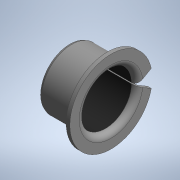
# Autodesk Inventor part: LFF-1410
Saved by Autodesk Inventor 2020.2 (Build 242310000, 310)
## iProperties
Part Number: LFF-1410
Material: 一般
Catalog Web Link: www.cadenas.de
Description: Flange Bushings-LFF
Vendor: OILES
Document SubType Name: Modeling
Designer: partserver
Manufacturer: OILES
Mass: 0.655588 g
Surface Area: 14.435 cm^2
Volume: 0.655588 cm^3
Density: 1 g/cm^3
Appearance: PSOLRGB-175-175-175
Category: PARTsolutions
Company: OILES
PSOL_IDENT_0: {$CADENAS_DATA\23d-libs\oiles\multi_bearings\oiles_drymet_lf\flange_bushings_lff.prj},166 {VTYP=3D},
PSOL_IDENT_1: {NB=LFF-1410},{LINA=LFF-1410},{NN=Flange Bushings},{DATE=15.04.2019 22:54:28},{GEOMDATE=27.10.2016 0
PSOL_IDENT_2: 4:28:40},{VERSION=},{LINEID=630},{WBVAR=},{WBNUMERIC=}  {NB=LFF-1410},{LINA=LFF-1410},{KT=DUMMY},{OR
PSOL_IDENT_3: DERNO=LFF-1410},{S=14},{SRT=-0.025/-0.043},{H=16.0},{HRT=H7(+0.018/0)},{ID=14},{IDR=+0.068/0},{OD=16
PSOL_IDENT_4: .0},{IDT=+0.065/+0.035},{T=1.0},{TT=0/-0.025},{F=22},{R=1.500},{FDT=0/-0.8},{FT=1.0},{FTT=0/-0.15},{
PSOL_IDENT_5: L=10},{LT=0/-0.3},{A=0.5},{AX=0.500},{B=C0.3},{BC=0.300},{TE=-200~+280°C},{P=49.0N/mm2 (500kgf/cm2)}
PSOL_IDENT_6: ,{V=0.65m/s (39m/min)},{PV=3.60N/mm2•m/s (2,200kgf/cm2•m/min)},{AIT=The I.D. tolerance after press f
PSOL_IDENT_7: itting is for reference only.},{AOT=Outer diameter is measrued by exclusive gauge.},{CAU=Please refe
PSOL_IDENT_8: r to catalog about detail.}
NB: LFF-1410
NN: Flange Bushings
NT: LFF
NBSYN: $ORDERNO.
LINA: LFF-1410
CATALOG: OILES CORPORATION
ORDERNO: LFF-1410
S: 14
SRT: -0.025/-0.043
H: 16
HRT: H7(+0.018/0)
ID: 14
IDR: +0.068/0
OD: 16
IDT: +0.065/+0.035
T: 1
TT: 0/-0.025
F: 22
FDT: 0/-0.8
FT: 1
FTT: 0/-0.15
L: 10
LT: 0/-0.3
TE: -200~+280°C
P: 49.0N/mm2 (500kgf/cm2)
V: 0.65m/s (39m/min)
PV: 3.60N/mm2•m/s (2,200kgf/cm2•m/min)
AIT: The I.D. tolerance after press fitting is for reference only.
AOT: Outer diameter is measrued by exclusive gauge.
CAU: Please refer to catalog about detail.
SUPPLIER: OILES
ARTICLENO: LFF-1410
BOMINFO: LFF-1410
CREATOR: CADENAS GmbH
Title: LFF-1410
Author: Cadenas PARTsolutions
Comments: LFF
Autodesk Inventor part; units mm, degrees
ref_plane "YZ Plane" through (0, 0, 0) normal (1, 0, 0) x (0, 1, 0)
ref_plane "XZ Plane" through (0, 0, 0) normal (0, 1, 0) x (-1, 0, 0)
ref_plane "XY Plane" through (0, 0, 0) normal (0, 0, 1) x (1, 0, 0)
sketch "Sketch_2" plane through (0, 0, 0) normal (0, 0, 1) x (1, 0, 0)
  line L0 (11, 0) -> (0, 0)
  arc A0 (0, 8.5) -> (1.5, 7) centre (1.5, 8.5) ccw
  line L1 (1.5, 7) -> (10.7, 7)
  line L2 (10.7, 7) -> (11, 7.3)
  line L3 (11, 7.3) -> (11, 7.818)
  line L4 (11, 7.818) -> (10.5, 8)
  line L5 (10.5, 8) -> (1.5, 8)
  arc A1 (1, 8.5) -> (1.5, 8) centre (1.5, 8.5) ccw
  line L6 (1, 8.5) -> (1, 11)
  line L7 (1, 11) -> (0, 11)
  line L8 (0, 11) -> (0, 8.5)
  dimension "d4" = 11
  constraints: 18 end point, 4 point on circle, 3 horizontal, 3 vertical, 2 centre point, 19 other
  measures "d4" distance between parallel lines of L8 L3
revolve "Revolution1" add sketch "Sketch_2" angle 360 about axis through (11, 0, 0) along (1, 0, 0)
sketch "Sketch_3" plane through (0, 0, 0) normal (1, 0, 0) x (0, 1, 0)
  line L0 (16.5263, 5.64) -> (6.7575, 0)
  line L1 (6.7575, 0) -> (16.5263, -5.64)
  line L2 (16.5263, -5.64) -> (16.5263, 5.64)
  constraints: 6 end point
extrude "Extrusion1" cut sketch "Sketch_3" along normal blind 11
body "Solid1"
